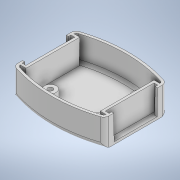
# Autodesk Inventor part: NVO_boat5
Saved by Autodesk Inventor 2020 (Build 240168000, 168)
## iProperties
Created: 2020-04-24
Part Number: NVO_boat5
Material: Generic
Document SubType Name: Modeling
Designer: nicva
Density: 1 g/cm^3
Appearance: Default
Author: nicva
Autodesk Inventor part; units mm, degrees
ref_plane "YZ Plane" through (0, 0, 0) normal (1, 0, 0) x (0, 1, 0)
ref_plane "XZ Plane" through (0, 0, 0) normal (0, 1, 0) x (-1, 0, 0)
ref_plane "XY Plane" through (0, 0, 0) normal (0, 0, 1) x (1, 0, 0)
sketch "Sketch1" plane through (0, 0, 0) normal (0, 1, 0) x (-1, 0, 0)
  line L0 (0, 0) -> (-54.991, 0)
  line L1 (-54.991, 0) -> (-54.991, -46.2026)
  line L2 (-54.991, -46.2026) -> (0, -46.2026)
  line L3 (0, -46.2026) -> (0, 0)
  line L4 (0, 0) -> (0, -4.7498)
  line L5 (0, -4.7498) -> (-54.991, -4.7498)
  line L6 (0, -46.2026) -> (0, -41.4528)
  line L7 (0, -41.4528) -> (-54.991, -41.4528)
  arc A0 (-54.991, -41.4528) -> (0, -41.4528) centre (-27.4955, 35.7549) ccw
  arc A1 (0, -4.7498) -> (-54.991, -4.7498) centre (-27.4955, -81.9575) ccw
  dimension "boat_l" = 54.991
  dimension "boat_w" = 46.2026
  dimension "d40" = 4.7498
  dimension "d41" = 54.991
  dimension "d42" = 4.7498
  dimension "d43" = 54.991
  constraints: 16 end point, 4 point on circle, 4 point on line, 3 perpendicular, 2 centre point, 1 horizontal, 1 tangent
  measures "boat_l" distance of L0.start L0.end
  measures "boat_w" distance of L0.end L1.end
  measures "d40" distance of L0.start L4.end
  measures "d41" distance of L4.end L5.end
  measures "d42" distance of L2.end L6.end
  measures "d43" distance of L6.end L7.end
extrude "Extrusion5" add sketch "Sketch1" along normal blind 15.0114 contours A1 L5 | L3 L7 L1 L5 | A0 L7
sketch "Sketch6" plane through (0, 0, 0) normal (0, -1, 0) x (1, 0, 0)
  line L0 (0, 0) -> (0, -10.1219)
  line L1 (0, -41.4528) -> (0, -4.7498) projected
  line L2 (0, -10.1219) -> (1.524, -10.1219)
  line L3 (1.524, -10.1219) -> (1.524, -8.5979)
  line L4 (1.524, -8.5979) -> (3.3782, -8.5979)
  line L5 (3.3782, -8.5979) -> (3.3782, -37.6047)
  line L6 (3.3782, -37.6047) -> (1.524, -37.6047)
  line L7 (1.524, -37.6047) -> (1.524, -36.0807)
  line L8 (1.524, -36.0807) -> (0, -36.0807)
  line L9 (0, -36.0807) -> (0, -10.1219)
  line L10 (0, 0) -> (54.991, 0)
  line L11 (54.991, 0) -> (54.991, -10.1219)
  line L12 (54.991, -4.7498) -> (54.991, -41.4528) projected
  line L13 (54.991, -10.1219) -> (53.467, -10.1219)
  line L14 (53.467, -10.1219) -> (53.467, -8.5979)
  line L15 (53.467, -8.5979) -> (51.6128, -8.5979)
  line L16 (51.6128, -8.5979) -> (51.6128, -37.6047)
  line L17 (51.6128, -37.6047) -> (53.467, -37.6047)
  line L18 (53.467, -37.6047) -> (53.467, -36.0807)
  line L19 (53.467, -36.0807) -> (54.991, -36.0807)
  line L20 (54.991, -10.1219) -> (54.991, -36.0807)
  dimension "thickness" = 1.524
  dimension "d53" = 10.1219
  dimension "d54" = 1.524
  dimension "d55" = 1.524
  dimension "d56" = 1.8542
  dimension "d57" = 29.0068
  dimension "d58" = 1.8542
  dimension "d59" = 1.524
  dimension "d60" = 1.524
  dimension "d61" = 54.991
  dimension "d62" = 10.1219
  dimension "d63" = 1.524
  dimension "d64" = 1.524
  dimension "d65" = 1.8542
  dimension "d66" = 29.0068
  dimension "d67" = 1.8542
  dimension "d68" = 1.524
  dimension "d69" = 1.524
  constraints: 38 end point, 8 point on line, 7 perpendicular, 2 horizontal, 1 collinear
  measures "d53" distance of L0.start L0.end
  measures "d54" distance of L0.end L2.end
  measures "d55" distance of L2.end L3.end
  measures "d56" distance of L3.end L4.end
  measures "d57" distance of L4.end L5.end
  measures "d58" distance of L5.end L6.end
  measures "d59" distance of L6.end L7.end
  measures "d60" distance of L7.end L8.end
  measures "d61" distance of L0.start L10.end
  measures "d62" distance of L10.end L11.end
  measures "d63" distance of L11.end L13.end
  measures "d64" distance of L13.end L14.end
  measures "d65" distance of L14.end L15.end
  measures "d66" distance of L15.end L16.end
  measures "d67" distance of L16.end L17.end
  measures "d68" distance of L17.end L18.end
  measures "d69" distance of L18.end L19.end
sketch "Sketch7" plane through (0, 0, 0) normal (0, -1, 0) x (1, 0, 0)
  line L0 (0, -4.7498) -> (0, -41.4528)
  line L1 (0, -41.4528) -> (0, -4.7498) projected
  line L2 (0, 0) -> (0, -4.7498)
  line L3 (0, -4.7498) -> (0, -41.4528)
  arc A0 (0, -41.4528) -> (54.991, -41.4528) centre (27.4955, 35.7549) ccw projected
  arc A1 (0, -41.4528) -> (54.991, -41.4528) centre (27.4955, 35.7549) ccw
  arc A2 (54.991, -4.7498) -> (0, -4.7498) centre (27.4955, -81.9575) ccw projected
  arc A3 (54.991, -4.7498) -> (0, -4.7498) centre (27.4955, -81.9575) ccw
  line L4 (54.991, -4.7498) -> (54.991, -41.4528) projected
  line L5 (54.991, -4.7498) -> (54.991, -41.4528)
  dimension "boat_w" = 46.2026
  dimension "fillet" = 4.7498
  dimension "d70" = 36.703
  dimension "d71" = 4.7498
  dimension "d72" = 36.703
  dimension "d73" = 36.703
  constraints: 8 end point, 4 point on circle, 2 centre point, 2 collinear, 1 vertical
  measures "d70" distance of L0.start L0.end
  measures "d71" distance of L2.start L0.start
  measures "d72" distance of L0.start L0.end
  measures "d73" distance of L4.start L4.end
extrude "Extrusion6" add sketch "Sketch7" along normal blind 1.524
fillet "Fillet5" radius 3.175 6 edges at (27.4955, -1.524, 0) (27.4955, -1.524, -46.2026) (54.991, 6.7437, -41.4528) (54.991, 6.7437, -4.7498) (0, 6.7437, -4.7498) (0, 6.7437, -41.4528)
extrude "Extrusion7" cut sketch "Sketch6" against normal blind 15.0114 draft 0.77
shell "Shell2" thickness 1.524 removed faces 1 at (38.8945, 15.0114, -28.003)
sketch "Sketch8" plane through (27.4955, 0, -81.9575) normal (0, 1, 0) x (1, 0, 0)
  line L0 (-27.4955, -81.9575) -> (-27.4955, -35.7549)
  line L1 (-27.4955, -71.8356) -> (-27.4955, -45.8768) projected
  line L2 (-27.4955, -35.7549) -> (-27.4955, -58.8562)
  line L3 (-27.4955, -58.8562) -> (0, -58.8562)
  line L4 (0, -58.8562) -> (-17.8435, -58.8562)
  line L5 (-17.8435, -58.8562) -> (-17.8435, -42.0287)
  line L6 (-17.8435, -42.0287) -> (17.8435, -42.0287)
  line L7 (17.8435, -42.0287) -> (17.8435, -75.6837)
  line L8 (17.8435, -75.6837) -> (-17.8435, -75.6837)
  line L9 (17.8435, -42.0287) -> (15.3035, -42.0287)
  line L10 (15.3035, -42.0287) -> (15.3035, -45.0767)
  circle A0 centre (15.3035, -45.0767) radius 1.5113
  circle A1 centre (15.3035, -45.0767) radius 3.5052
  line L11 (15.3035, -45.0767) -> (15.3035, -68.5717)
  line L12 (15.3035, -68.5717) -> (-14.1605, -68.5717)
  circle A2 centre (-14.1605, -68.5717) radius 1.5113
  circle A3 centre (-14.1605, -68.5717) radius 3.5052
  circle A4 centre (15.3035, -68.5717) radius 1.5113
  circle A5 centre (15.3035, -68.5717) radius 3.5052
  line L13 (15.3035, -68.5717) -> (15.3035, -78.9262)
  line L14 (-17.8435, -58.8562) -> (-22.3914, -58.8562)
  line L15 (-22.3914, -75.0855) -> (-22.3914, -42.6269) projected
  dimension "d80" = 46.2026
  dimension "d81" = 23.1013
  dimension "d82" = 27.4955
  dimension "d83" = 17.8435
  dimension "d84" = 16.8275
  dimension "d86" = 33.655
  dimension "d87" = 35.687
  dimension "d88" = 2.54
  dimension "d89" = 3.048
  dimension "d92" = 23.495
  dimension "d93" = 29.464
  dimension "d94" = 3.0226
  dimension "d95" = 7.0104
  dimension "d100" = 10.3546
  dimension "d101" = 4.5479
  constraints: 28 end point, 6 centre point, 6 coincident, 6 perpendicular, 3 point on line, 2 midpoint, 2 vertical, 1 collinear
  measures "d80" distance of L0.start L0.end
  measures "d81" distance of L0.end L2.end
  measures "d82" distance of L2.end L3.end
  measures "d83" distance of L3.end L4.end
  measures "d84" distance of L4.end L5.end
  measures "d86" distance of L6.end L7.end
  measures "d87" distance of L7.end L8.end
  measures "d88" distance of L6.end L9.end
  measures "d89" distance of L9.end L10.end
  measures "d92" distance of L11.start L11.end
  measures "d93" distance of L11.end L12.end
  measures "d94" diameter of A2
  measures "d95" diameter of A3
  measures "d100" distance of L13.start L13.end
  measures "d101" distance of L14.end L4.end
extrude "Extrusion8" add sketch "Sketch8" along normal blind 5.0038 contours A1 L6 | L6 L10 A0 L11 A1 | L6 A1 L7 L11 A0 L10 | A1 L7 | A5 L7 L13 A4 L11 | L11 A4 L12 A5 | A5 L7 | L12 A4 L13 A5 | A3
equation "\"boat_l\" = length + 4 * thickness + 2 * fillet + 2 * mount_w"
equation "\"boat_w\" = extra + 2 * fillet + 2 * thickness"
equation "\"d40\" = fillet"
equation "\"d41\" = boat_l"
equation "\"d42\" = fillet"
equation "\"d43\" = boat_l"
equation "\"d51\" = height"
equation "\"thickness\" = 1.524"
equation "\"d53\" = thickness + 0.5 * boat_w - 0.5 * mount_l"
equation "\"d54\" = thickness"
equation "\"d55\" = thickness"
equation "\"d56\" = mount_w"
equation "\"d57\" = mount_l"
equation "\"d58\" = mount_w"
equation "\"d59\" = thickness"
equation "\"d60\" = thickness"
equation "\"d61\" = boat_l"
equation "\"d62\" = thickness + 0.5 * boat_w - 0.5 * mount_l"
equation "\"d63\" = thickness"
equation "\"d64\" = thickness"
equation "\"d65\" = mount_w"
equation "\"d66\" = mount_l"
equation "\"d67\" = mount_w"
equation "\"d68\" = thickness"
equation "\"d69\" = thickness"
equation "\"fillet\" = 4.7498"
equation "\"d70\" = boat_w - 2 * fillet"
equation "\"d71\" = fillet"
equation "\"d72\" = boat_w - 2 * fillet"
equation "\"d73\" = boat_w - 2 * fillet"
equation "\"d74\" = thickness"
equation "\"d77\" = height"
equation "\"d79\" = thickness"
equation "\"d80\" = boat_w"
equation "\"d81\" = 0.5 * boat_w"
equation "\"d82\" = 0.5 * boat_l"
equation "\"d83\" = 0.5 * length"
equation "\"d84\" = 0.5 * extra"
equation "\"d86\" = extra"
equation "\"d87\" = length"
equation "\"d88\" = edge_l"
equation "\"d89\" = edge_w"
equation "\"d92\" = screw_w"
equation "\"d93\" = screw_l"
equation "\"d94\" = threads"
equation "\"d95\" = standoff"
equation "\"d98\" = screw"
equation "\"screw\" = 5.0038"
equation "\"length\" = 35.687"
equation "\"width\" = 44.323"
equation "\"ideal\" = 28.575"
equation "\"extra\" = 33.655"
equation "\"mount_l\" = 29.0068"
equation "\"mount_w\" = 1.8542"
equation "\"threads\" = 3.0226"
equation "\"edge_w\" = 3.048"
equation "\"edge_l\" = 2.54"
equation "\"screw_w\" = 23.495"
equation "\"screw_l\" = 29.464"
equation "\"height\" = 15.0114"
equation "\"standoff\" = 7.0104"
body "Solid2"
